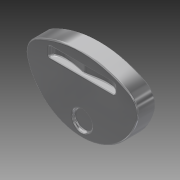
# Autodesk Inventor part: Bottom - Anvil
Saved by Autodesk Inventor 2011 (Build 150239000, 239)
## iProperties
Company: Autodesk
Shininess: 64.0
Length Units: 11272
Angle Units: 11279
Time Units: 11290
Mass Units: 11286
Length Display Precision: 3
Angle Display Precision: 2
Compacted: True
Part Number: Bottom - Anvil
Document SubType Name: Modeling
Created: 2002-09-26
Designer: Autodesk, Inc.
Material: Stainless Steel, Austenitic
Project: Inventor Samples
Density: 8.03 g/cm^3
Mass: 4.15498 g
Surface Area: 4.9256 cm^2
Volume: 0.517432 cm^3
Density: 0.0
Volumn: 0.0
Area: 0.0
PropertySet Name: Model Information
Control State: 0
Master: False
Checked Out: False
Author: Autodesk, Inc.
Revision Number: A
Autodesk Inventor part; units mm, degrees
ref_plane "YZ Plane" through (0, 0, 0) normal (1, 0, 0) x (0, 1, 0)
ref_plane "XZ Plane" through (0, 0, 0) normal (0, 1, 0) x (-1, 0, 0)
sketch "Sketch1" plane through (0, 0, 0) normal (0, 0, 1) x (1, 0, 0)
  arc A0 (-7.6855, 4.8772) -> (-9.2225, 1.3053) centre (-6.1484, 2.0991) ccw projected
  arc A1 (-9.2225, 1.3053) -> (9.2225, 1.3053) centre (0, 3.6866) ccw projected
  arc A2 (9.2225, 1.3053) -> (7.6855, 4.8772) centre (6.1484, 2.0991) ccw projected
  arc A3 (7.6855, 4.8772) -> (-7.6855, 4.8772) centre (0, -9.0134) ccw projected
  arc A4 (-8.9766, 1.3688) -> (8.9766, 1.3688) centre (0, 3.6866) ccw
  arc A5 (-7.5625, 4.655) -> (-8.9766, 1.3688) centre (-6.1484, 2.0991) ccw
  arc A6 (7.5625, 4.655) -> (-7.5625, 4.655) centre (0, -9.0134) ccw
  arc A7 (8.9766, 1.3688) -> (7.5625, 4.655) centre (6.1484, 2.0991) ccw
  dimension "d19" = 0.254
  constraints: 8 point on circle, 4 centre point, 3 other
  measures "d19" radial gap between concentric circles of A7 A2
extrude "Extrusion1" add sketch "Sketch1" along normal blind 3.175 contours A5 A6 A7 A4
sketch "Sketch2" plane through (0, 0, 3.175) normal (0, 0, 1) x (1, 0, 0)
  line L0 (0, 9.046) -> (0, -8.0228) projected
  circle A0 centre (0, -3.175) radius 1.5875
  line L1 (-12.6971, 0) -> (12.6971, 0) projected
  dimension "d3" = 3.175
  dimension "d4" = 3.175
  constraints: 1 centre point, 1 point on line
  measures "d3" distance from line of A0.centre L1
  measures "d4" diameter of A0
extrude "Extrusion2" cut sketch "Sketch2" against normal blind 0.508
fillet "Fillet1" radius 0.254 2 edges at (-1.5875, -3.175, 3.175) (-1.5875, -3.175, 2.667)
chamfer "Chamfer1" distance 0.381 angle 45 4 edges at (0, 6.6076, 0) (8.8315, 3.2537, 0) (0, -5.5844, 0) (-8.8315, 3.2537, 0)
ref_plane "Work Plane1" through (0, 3.9624, 0) normal (0, 1, 0) x (-1, 0, 0)
sketch "Sketch3" plane through (0, 3.9624, 0) normal (0, 1, 0) x (-1, 0, 0)
  line L0 (-8.9766, 3.175) -> (8.9766, 3.175) projected
  line L1 (0, 1.6708) -> (0, 3.4402) projected
  spline S0 degree 2 poles (-5.4429, 3.175) (-5.1658, 1.4753) (0, 2.667) knots 0 0 0 1 1 1
  line L2 (-5.4429, 3.175) -> (0, 3.175)
  line L3 (0, 2.667) -> (0, 3.175)
  point P0 (-4.7752, 2.3876)
  dimension "d11" = 0.7874
  dimension "d12" = 4.7752
  dimension "d18" = 0.508
  constraints: 4 end point, 3 point on line, 1 midpoint, 1 perpendicular, 3 other
  measures "d11" distance from line of L0 point (-4.775, 2.388)
  measures "d12" distance from line of L1 point (-4.775, 2.388)
  measures "d18" distance of L3.start L2.end
extrude "Extrusion3" cut sketch "Sketch3" against normal mid plane 1.524
mirror "Mirror1" about plane through (0, 0, 0) normal (1, 0, 0) of "Extrusion3"
fillet "Fillet2" radius 1.524 2 edges at (0, 3.5814, 2.667) (0, 4.3434, 2.667)
fillet "Fillet3" radius 0.254 4 edges at (4.0297, 4.7244, 2.207) (-4.0297, 4.7244, 2.207) (4.0297, 3.2004, 2.207) (-4.0297, 3.2004, 2.207)
fillet "Fillet4" radius 0.254 10 edges at (5.4429, 3.7084, 3.175) (5.4429, 4.2164, 3.175) (5.3674, 3.2748, 3.175) (0, 3.2004, 3.175) (-5.3674, 3.2748, 3.175) (-5.3674, 4.65, 3.175) (-5.4429, 3.7084, 3.175) (-5.4429, 4.2164, 3.175) (5.3674, 4.65, 3.175) (0, 4.7244, 3.175)
fillet "Fillet5" radius 0.254 4 edges at (0, 6.6076, 3.175) (8.8315, 3.2537, 3.175) (0, -5.5844, 3.175) (-8.8315, 3.2537, 3.175)
body "Solid1"
